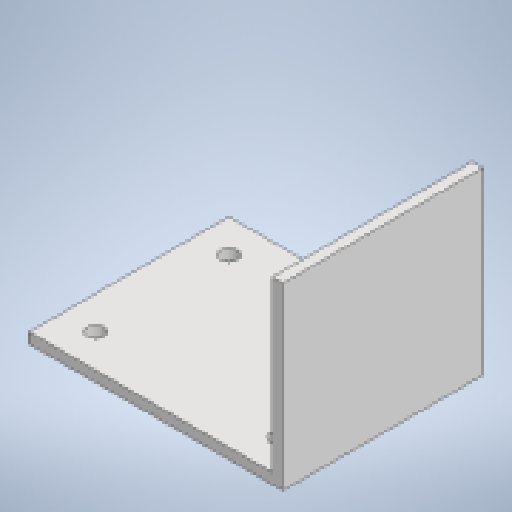
# Autodesk Inventor part: Z_Screw_Holder_Bracket
Saved by Autodesk Inventor 2023 (Build 270158000, 158)
## iProperties
Created: 2022-05-06
Part Number: Z_Screw_Holder_Bracket
Material: Generic
Document SubType Name: Modeling
Designer: plebbb
Density: 1 g/cm^3
Appearance: Default
Author: plebbb
Autodesk Inventor part; units mm, degrees
ref_plane "YZ Plane" through (0, 0, 0) normal (1, 0, 0) x (0, 1, 0)
ref_plane "XZ Plane" through (0, 0, 0) normal (0, 1, 0) x (-1, 0, 0)
ref_plane "XY Plane" through (0, 0, 0) normal (0, 0, 1) x (1, 0, 0)
sketch "Sketch1" plane through (0, 0, 0) normal (0, 0, 1) x (1, 0, 0)
  line L0 (0, 0) -> (-76.2, 0)
  line L1 (-76.2, 0) -> (-76.2, 3.175)
  line L2 (-76.2, 3.175) -> (-3.175, 3.175)
  line L3 (-3.175, 3.175) -> (-3.175, 53.975)
  line L4 (-3.175, 53.975) -> (0, 53.975)
  line L5 (0, 53.975) -> (0, 0)
  dimension "d0" = 76.2
  dimension "d1" = 50.8
  dimension "d2" = 3.175
  constraints: 12 end point, 4 perpendicular, 1 horizontal, 1 parallel, 1 vertical
  measures "d0" distance of L0.start L0.end
  measures "d1" distance of L2.end L3.end
  measures "d2" distance of L0.end L1.end
extrude "Extrusion1" add sketch "Sketch1" along normal blind 60
sketch "Sketch2" plane through (-76.2, 3.175, 0) normal (0, 1, 0) x (1, 0, 0)
  line L0 (10.98, -50) -> (63.98, -50) construction
  line L1 (63.98, -50) -> (63.98, -10) construction
  line L2 (63.98, -10) -> (10.98, -10) construction
  line L3 (10.98, -10) -> (10.98, -50) construction
  line L4 (0, 0) -> (0, -60) construction
  line L5 (76.2, 0) -> (76.2, -60) construction
  circle A0 centre (10.98, -50) radius 2.5
  circle A1 centre (10.98, -10) radius 2.5
  circle A2 centre (63.98, -50) radius 2.5
  circle A3 centre (63.98, -10) radius 2.5
  point P0 (0, -30)
  point P1 (10.98, -30)
  dimension "d5" = 12.22
  dimension "d6" = 53
  dimension "d7" = 40
  dimension "d8" = 5
  constraints: 8 end point, 4 centre point, 4 coincident, 3 equal radius, 2 midpoint, 2 parallel, 1 horizontal, 1 horizontal alignment, 1 perpendicular
  measures "d5" distance between parallel lines of L1 L5
  measures "d6" distance of L0.start L0.end
  measures "d7" distance of L2.end L0.start
  measures "d8" diameter of A0
extrude "Extrusion2" cut sketch "Sketch2" against normal blind 60
body "Solid1"
